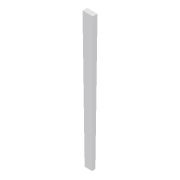
# Autodesk Inventor part: molecularBeam
Saved by Autodesk Inventor 2015 SP1 (Build 190203100, 203)
## iProperties
Created: 2016-10-10
Part Number: molecularBeam
Material: Generic
Document SubType Name: Modeling
Designer: I Rabey
Density: 1 g/cm^3
Appearance: Default
Author: I Rabey
Autodesk Inventor part; units mm, degrees
ref_plane "YZ Plane" through (0, 0, 0) normal (1, 0, 0) x (0, 1, 0)
ref_plane "XY Plane" through (0, 0, 0) normal (0, 0, 1) x (1, 0, 0)
sketch "Sketch1" plane through (0, 0, 0) normal (0, 1, 0) x (-1, 0, 0)
  line L0 (13.15, 6) -> (-13.15, 6)
  line L1 (-13.15, 6) -> (-13.15, -6)
  line L2 (-13.15, -6) -> (13.15, -6)
  line L3 (13.15, -6) -> (13.15, 6)
  line L4 (13.15, 6) -> (-13.15, -6) construction
  line L5 (-13.15, 6) -> (13.15, -6) construction
  point P0 (0, 0)
  dimension "d0" = 26.3
  dimension "d1" = 12
  constraints: 12 end point, 2 midpoint, 2 parallel, 1 horizontal, 1 perpendicular
  measures "d0" distance of L2.end L1.end
  measures "d1" distance of L1.end L0.end
ref_plane "Work Plane1" through (0, 480, 0) normal (0, 1, 0) x (-1, 0, 0)
sketch "Sketch2" plane through (0, 480, 0) normal (0, 1, 0) x (-1, 0, 0)
  line L0 (-18.25, 8.35) -> (18.25, 8.35)
  line L1 (18.25, 8.35) -> (18.25, -8.35)
  line L2 (18.25, -8.35) -> (-18.25, -8.35)
  line L3 (-18.25, -8.35) -> (-18.25, 8.35)
  line L4 (-18.25, 8.35) -> (18.25, -8.35) construction
  line L5 (18.25, 8.35) -> (-18.25, -8.35) construction
  point P0 (0, 0)
  dimension "d3" = 36.5
  dimension "d4" = 16.7
  constraints: 12 end point, 2 midpoint, 2 parallel, 1 horizontal, 1 perpendicular
  measures "d3" distance of L1.end L2.end
  measures "d4" distance of L0.end L1.end
loft "Loft1" add profiles "Sketch1", "Sketch2"
body "Solid1"
